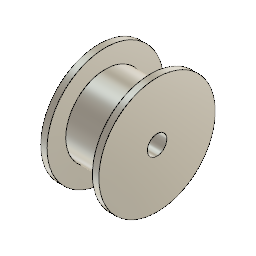
y_idler_tensioner_e3d (Autodesk Fusion 360 archive; units mm, degrees)
design "2gt_idler_20t_6mmbelt"
Autodesk Fusion 360 part; units mm, degrees
sketch "Sketch1" plane through (0, 0, 0) normal (1, 0, 0) x (0, 1, 0)
  circle A0 centre (0, 0) radius 6.11
  circle A1 centre (0, 0) radius 9
  circle A2 centre (0, 0) radius 1.5
  circle A3 centre (0, 0) radius 6.365 construction
  dimension "d1" = 3
  dimension "d2" = 12.22
  dimension "d3" = 18
  dimension "d11" = 12.73
  measures "d1" diameter of A2
  measures "d2" diameter of A0
  measures "d3" diameter of A1
  measures "d11" diameter of A3
extrude "Extrude1" add sketch "Sketch1" along normal blind 9 contours A0 | A1
extrude "Extrude2" cut sketch "Sketch1" along normal blind 7 from surface at 1 contours A1
equation "d2 = outside_dia"
equation "pitch_dia = 12.73 mm"
equation "outside_dia = 12.22 mm"
equation "d11 = pitch_dia"
